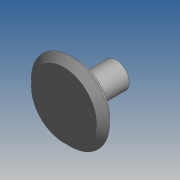
# Autodesk Inventor part: P006-Soupape_entree
Saved by Autodesk Inventor 2021.4 (Build 254397000, 397)
## iProperties
Created: 2022-03-24
Part Number: P006-Soupape_entree
Material: Générique
Document SubType Name: Modeling
Designer: Maintenant Prêt
Density: 1 g/cm^3
Appearance: Par défaut
Author: Maintenant Prêt
Autodesk Inventor part; units mm, degrees
ref_plane "YZ Plane" through (0, 0, 0) normal (1, 0, 0) x (0, 1, 0)
ref_plane "XZ Plane" through (0, 0, 0) normal (0, 1, 0) x (-1, 0, 0)
ref_plane "XY Plane" through (0, 0, 0) normal (0, 0, 1) x (1, 0, 0)
sketch "Sketch2" plane through (0, 0, 0) normal (0, 0, 1) x (1, 0, 0)
  line L0 (0, -1.6) -> (0, 9.6) construction
  line L1 (-7.2, 0) -> (1.2, 0) construction
  line L2 (0, 0) -> (-6, 0)
  line L3 (-6, 2) -> (-2, 2)
  line L4 (-2, 2) -> (-2, 4.114)
  line L5 (-2, 4.7135) -> (-2, 8)
  line L6 (-2, 8) -> (0, 8)
  line L7 (0, 0) -> (-6, 0)
  line L8 (-6, 2) -> (-6, 0)
  line L9 (-2, 3.3248) -> (-2, 5.5716)
  line L10 (0, 8) -> (0, 0)
  dimension "d0" = 2
  dimension "d1" = 6
  dimension "d3" = 2
  dimension "d4" = 8
  constraints: 18 end point, 6 point on line, 4 perpendicular, 1 horizontal, 1 parallel
  measures "d0" distance between parallel lines of L5 L0
  measures "d1" distance between parallel lines of L8 L0
  measures "d3" distance between parallel lines of L1 L3
  measures "d4" distance between parallel lines of L1 L6
revolve "Revolution1" add sketch "Sketch2" angle 360 about axis through (0, -10, 0) along (0, 1, 0)
chamfer "Chamfer1" distance 1 angle 45 1 edges at (6, 2, 0)
chamfer "Chamfer2" distance 1 angle 45 1 edges at (6, 0, 0)
body "Solid1"
